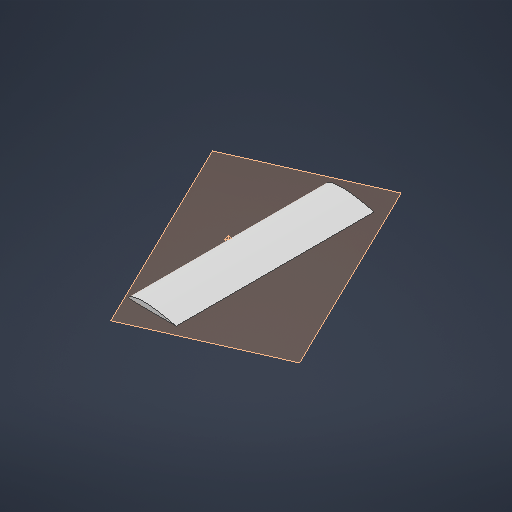
# Autodesk Inventor part: Airfoil
Saved by Autodesk Inventor 2026.1 (Build 301233000, 233)
## iProperties
Created: 2026-06-28
Part Number: Airfoil
Material: Generic
Document SubType Name: Modeling
Designer: adria
Density: 1 g/cm^3
Appearance: Default
Author: adria
Autodesk Inventor part; units mm, degrees
ref_plane "YZ Plane" through (0, 0, 0) normal (1, 0, 0) x (0, 1, 0)
ref_plane "XZ Plane" through (0, 0, 0) normal (0, 1, 0) x (-1, 0, 0)
ref_plane "XY Plane" through (0, 0, 0) normal (0, 0, 1) x (1, 0, 0)
sketch "Airfoil" plane through (0, 0, 0) normal (0, 0, 1) x (1, 0, 0)
  spline S0 degree 3 poles (360.0001, -3.1258) (359.9999, -3.1093) (358.5352, -2.9642) (357.0563, -2.6727) (353.499, -2.1006) (349.1715, -1.2943) (343.5455, -0.2589) (336.9185, 1.0019) (329.2813, 2.4997) (320.7437, 4.2061) (311.3885, 6.1167) (301.3069, 8.1831) (290.5978, 10.3802) (279.3545, 12.6643) (267.6408, 14.9381) (255.5164, 17.1385) (243.0539, 19.2958) (230.3132, 21.3308) (217.3729, 23.2252) (204.3064, 24.9736) (191.1725, 26.4966) (178.0452, 27.8241) (164.9837, 28.9046) (152.0591, 29.712) (139.3323, 30.2778) (126.8644, 30.5476) (114.7179, 30.5317) (102.9483, 30.2384) (91.6056, 29.6426) (80.7401, 28.7689) (70.3983, 27.6332) (60.634, 26.2223) (51.4811, 24.5969) (42.9826, 22.7423) (35.1746, 20.693) (28.0854, 18.4861) (21.7475, 16.1422) (16.1794, 13.7122) (11.405, 11.2286) (7.4429, 8.7282) (4.3064, 6.298) (1.9678, 3.9602) (0.5759, 1.8788) (-0.2825, -0.1229) (0.8182, -1.9616) (2.9085, -3.1846) (5.9423, -4.3926) (10.0909, -5.2147) (15.3188, -5.8919) (21.6524, -6.4415) (29.0414, -6.8802) (37.4377, -7.2114) (46.7843, -7.4502) (57.0133, -7.6106) (68.0506, -7.6971) (79.8194, -7.7126) (92.2551, -7.6326) (105.2911, -7.4608) (118.8533, -7.2529) (132.849, -7.0142) (147.1809, -6.7663) (161.7434, -6.5195) (176.4331, -6.2697) (191.1431, -6.0148) (205.7764, -5.7632) (220.2333, -5.52) (234.4223, -5.2741) (248.2526, -5.0368) (261.628, -4.8128) (274.4379, -4.5908) (286.5696, -4.3821) (297.9608, -4.1861) (308.5993, -4.0068) (318.4689, -3.8376) (327.5045, -3.6854) (335.6112, -3.5403) (342.6591, -3.4259) (348.6433, -3.3202) (353.2298, -3.2392) (356.964, -3.1905) (358.5007, -3.1269) (360.0002, -3.1425) (360.0001, -3.1258) knots 0 0 0 0 0.000951 0.003756 0.008317 0.014521 0.022293 0.03156 0.04222 0.054151 0.067231 0.081331 0.096307 0.112011 0.128327 0.145184 0.162487 0.180134 0.198032 0.216058 0.234133 0.25219 0.270102 0.287815 0.305233 0.322283 0.338894 0.354984 0.370504 0.385415 0.39963 0.413113 0.42582 0.437701 0.448735 0.458877 0.468103 0.476402 0.483746 0.490131 0.495554 0.500009 0.503513 0.506003 0.508226 0.511498 0.515852 0.521548 0.528758 0.537453 0.547579 0.559078 0.571871 0.585877 0.600983 0.617084 0.634085 0.651924 0.670487 0.689646 0.709262 0.729203 0.749306 0.769443 0.789468 0.809256 0.828671 0.847599 0.865917 0.883468 0.900079 0.915619 0.930136 0.943664 0.956051 0.96716 0.976853 0.984996 0.991473 0.996184 0.999041 1 1 1 1
  line L0 (360.0001, -3.1258) -> (359.9999, -3.1093) construction
  line L1 (359.9999, -3.1093) -> (358.5352, -2.9642) construction
  line L2 (358.5352, -2.9642) -> (357.0563, -2.6727) construction
  line L3 (357.0563, -2.6727) -> (353.499, -2.1006) construction
  line L4 (353.499, -2.1006) -> (349.1715, -1.2943) construction
  line L5 (349.1715, -1.2943) -> (343.5455, -0.2589) construction
  line L6 (343.5455, -0.2589) -> (336.9185, 1.0019) construction
  line L7 (336.9185, 1.0019) -> (329.2813, 2.4997) construction
  line L8 (329.2813, 2.4997) -> (320.7437, 4.2061) construction
  line L9 (320.7437, 4.2061) -> (311.3885, 6.1167) construction
  line L10 (311.3885, 6.1167) -> (301.3069, 8.1831) construction
  line L11 (301.3069, 8.1831) -> (290.5978, 10.3802) construction
  line L12 (290.5978, 10.3802) -> (279.3545, 12.6643) construction
  line L13 (279.3545, 12.6643) -> (267.6408, 14.9381) construction
  line L14 (267.6408, 14.9381) -> (255.5164, 17.1385) construction
  line L15 (255.5164, 17.1385) -> (243.0539, 19.2958) construction
  line L16 (243.0539, 19.2958) -> (230.3132, 21.3308) construction
  line L17 (230.3132, 21.3308) -> (217.3729, 23.2252) construction
  line L18 (217.3729, 23.2252) -> (204.3064, 24.9736) construction
  line L19 (204.3064, 24.9736) -> (191.1725, 26.4966) construction
  line L20 (191.1725, 26.4966) -> (178.0452, 27.8241) construction
  line L21 (178.0452, 27.8241) -> (164.9837, 28.9046) construction
  line L22 (164.9837, 28.9046) -> (152.0591, 29.712) construction
  line L23 (152.0591, 29.712) -> (139.3323, 30.2778) construction
  line L24 (139.3323, 30.2778) -> (126.8644, 30.5476) construction
  line L25 (126.8644, 30.5476) -> (114.7179, 30.5317) construction
  line L26 (114.7179, 30.5317) -> (102.9483, 30.2384) construction
  line L27 (102.9483, 30.2384) -> (91.6056, 29.6426) construction
  line L28 (91.6056, 29.6426) -> (80.7401, 28.7689) construction
  line L29 (80.7401, 28.7689) -> (70.3983, 27.6332) construction
  line L30 (70.3983, 27.6332) -> (60.634, 26.2223) construction
  line L31 (60.634, 26.2223) -> (51.4811, 24.5969) construction
  line L32 (51.4811, 24.5969) -> (42.9826, 22.7423) construction
  line L33 (42.9826, 22.7423) -> (35.1746, 20.693) construction
  line L34 (35.1746, 20.693) -> (28.0854, 18.4861) construction
  line L35 (28.0854, 18.4861) -> (21.7475, 16.1422) construction
  line L36 (21.7475, 16.1422) -> (16.1794, 13.7122) construction
  line L37 (16.1794, 13.7122) -> (11.405, 11.2286) construction
  line L38 (11.405, 11.2286) -> (7.4429, 8.7282) construction
  line L39 (7.4429, 8.7282) -> (4.3064, 6.298) construction
  line L40 (4.3064, 6.298) -> (1.9678, 3.9602) construction
  line L41 (1.9678, 3.9602) -> (0.5759, 1.8788) construction
  line L42 (0.5759, 1.8788) -> (-0.2825, -0.1229) construction
  line L43 (-0.2825, -0.1229) -> (0.8182, -1.9616) construction
  line L44 (0.8182, -1.9616) -> (2.9085, -3.1846) construction
  line L45 (2.9085, -3.1846) -> (5.9423, -4.3926) construction
  line L46 (5.9423, -4.3926) -> (10.0909, -5.2147) construction
  line L47 (10.0909, -5.2147) -> (15.3188, -5.8919) construction
  line L48 (15.3188, -5.8919) -> (21.6524, -6.4415) construction
  line L49 (21.6524, -6.4415) -> (29.0414, -6.8802) construction
  line L50 (29.0414, -6.8802) -> (37.4377, -7.2114) construction
  line L51 (37.4377, -7.2114) -> (46.7843, -7.4502) construction
  line L52 (46.7843, -7.4502) -> (57.0133, -7.6106) construction
  line L53 (57.0133, -7.6106) -> (68.0506, -7.6971) construction
  line L54 (68.0506, -7.6971) -> (79.8194, -7.7126) construction
  line L55 (79.8194, -7.7126) -> (92.2551, -7.6326) construction
  line L56 (92.2551, -7.6326) -> (105.2911, -7.4608) construction
  line L57 (105.2911, -7.4608) -> (118.8533, -7.2529) construction
  line L58 (118.8533, -7.2529) -> (132.849, -7.0142) construction
  line L59 (132.849, -7.0142) -> (147.1809, -6.7663) construction
  line L60 (147.1809, -6.7663) -> (161.7434, -6.5195) construction
  line L61 (161.7434, -6.5195) -> (176.4331, -6.2697) construction
  line L62 (176.4331, -6.2697) -> (191.1431, -6.0148) construction
  line L63 (191.1431, -6.0148) -> (205.7764, -5.7632) construction
  line L64 (205.7764, -5.7632) -> (220.2333, -5.52) construction
  line L65 (220.2333, -5.52) -> (234.4223, -5.2741) construction
  line L66 (234.4223, -5.2741) -> (248.2526, -5.0368) construction
  line L67 (248.2526, -5.0368) -> (261.628, -4.8128) construction
  line L68 (261.628, -4.8128) -> (274.4379, -4.5908) construction
  line L69 (274.4379, -4.5908) -> (286.5696, -4.3821) construction
  line L70 (286.5696, -4.3821) -> (297.9608, -4.1861) construction
  line L71 (297.9608, -4.1861) -> (308.5993, -4.0068) construction
  line L72 (308.5993, -4.0068) -> (318.4689, -3.8376) construction
  line L73 (318.4689, -3.8376) -> (327.5045, -3.6854) construction
  line L74 (327.5045, -3.6854) -> (335.6112, -3.5403) construction
  line L75 (335.6112, -3.5403) -> (342.6591, -3.4259) construction
  line L76 (342.6591, -3.4259) -> (348.6433, -3.3202) construction
  line L77 (348.6433, -3.3202) -> (353.2298, -3.2392) construction
  line L78 (353.2298, -3.2392) -> (356.964, -3.1905) construction
  line L79 (356.964, -3.1905) -> (358.5007, -3.1269) construction
  line L80 (358.5007, -3.1269) -> (360.0002, -3.1425) construction
  line L81 (360.0002, -3.1425) -> (360.0001, -3.1258) construction
  line L82 (0, 0) -> (360.0001, -3.1258) construction
  point P0 (179.3364, 5.2593)
sketch "Sketch1" plane through (0, 0, 0) normal (0, 0, 1) x (1, 0, 0)
  line L0 (0, 0) -> (0, -30) construction
  line L1 (0, -30) -> (300, -30) construction
  spline S0 degree 3 poles (359.8903, -9.4241) (359.8904, -9.4075) (358.4284, -9.2368) (356.9549, -8.9194) (353.4081, -8.2852) (349.0954, -7.4034) (343.4884, -6.2696) (336.8844, -4.8931) (329.2747, -3.2619) (320.7682, -1.4064) (311.4479, 0.6676) (301.4039, 2.91) (290.7349, 5.2942) (279.5333, 7.7746) (267.8612, 10.2531) (255.7771, 12.6653) (243.3543, 15.0402) (230.6512, 17.2979) (217.746, 19.4184) (204.712, 21.3951) (191.6068, 23.1477) (178.5047, 24.7047) (165.4642, 26.0136) (152.5557, 27.047) (139.8408, 27.8354) (127.3795, 28.3233) (115.2345, 28.5198) (103.4616, 28.4326) (92.1102, 28.0353) (81.2311, 27.3519) (70.8711, 26.3973) (61.0835, 25.1574) (51.9036, 23.6924) (43.374, 21.9868) (35.5313, 20.0744) (28.4046, 17.9919) (22.0266, 15.7592) (16.4168, 13.427) (11.5997, 11.0273) (7.5944, 8.5967) (4.4159, 6.2217) (2.0368, 3.9251) (0.6086, 1.8684) (-0.2846, -0.1179) (0.7837, -1.9756) (2.8523, -3.235) (5.8645, -4.4959) (9.9981, -5.3905) (15.2134, -6.159) (21.5363, -6.8193) (28.9165, -7.3873) (37.3058, -7.8653) (46.6468, -8.2676) (56.8714, -8.607) (67.9055, -8.8866) (79.6723, -9.108) (92.1074, -9.2455) (105.1444, -9.3019) (118.7082, -9.3313) (132.7059, -9.3375) (147.04, -9.3404) (161.6045, -9.3484) (176.2964, -9.3557) (191.0086, -9.3582) (205.644, -9.3627) (220.103, -9.3725) (234.2942, -9.3748) (248.1264, -9.3796) (261.5037, -9.3896) (274.3155, -9.3917) (286.4491, -9.3953) (297.842, -9.3987) (308.4819, -9.4056) (318.353, -9.4091) (327.3899, -9.415) (335.4978, -9.4117) (342.5467, -9.4207) (348.5319, -9.4197) (353.1191, -9.4189) (356.8535, -9.4356) (358.3911, -9.3989) (359.8902, -9.4407) (359.8903, -9.4241) knots 0 0 0 0 0.000951 0.003756 0.008317 0.014521 0.022293 0.03156 0.04222 0.054151 0.067231 0.081331 0.096307 0.112011 0.128327 0.145184 0.162487 0.180134 0.198032 0.216058 0.234133 0.25219 0.270102 0.287815 0.305233 0.322283 0.338894 0.354984 0.370504 0.385415 0.39963 0.413113 0.42582 0.437701 0.448735 0.458877 0.468103 0.476402 0.483746 0.490131 0.495554 0.500009 0.503513 0.506003 0.508226 0.511498 0.515852 0.521548 0.528758 0.537453 0.547579 0.559078 0.571871 0.585877 0.600983 0.617084 0.634085 0.651924 0.670487 0.689646 0.709262 0.729203 0.749306 0.769443 0.789468 0.809256 0.828671 0.847599 0.865917 0.883468 0.900079 0.915619 0.930136 0.943664 0.956051 0.96716 0.976853 0.984996 0.991473 0.996184 0.999041 1 1 1 1
  line L2 (359.8903, -9.4241) -> (359.8904, -9.4075) construction
  line L3 (359.8904, -9.4075) -> (358.4284, -9.2368) construction
  line L4 (358.4284, -9.2368) -> (356.9549, -8.9194) construction
  line L5 (356.9549, -8.9194) -> (353.4081, -8.2852) construction
  line L6 (353.4081, -8.2852) -> (349.0954, -7.4034) construction
  line L7 (349.0954, -7.4034) -> (343.4884, -6.2696) construction
  line L8 (343.4884, -6.2696) -> (336.8844, -4.8931) construction
  line L9 (336.8844, -4.8931) -> (329.2747, -3.2619) construction
  line L10 (329.2747, -3.2619) -> (320.7682, -1.4064) construction
  line L11 (320.7682, -1.4064) -> (311.4479, 0.6676) construction
  line L12 (311.4479, 0.6676) -> (301.4039, 2.91) construction
  line L13 (301.4039, 2.91) -> (290.7349, 5.2942) construction
  line L14 (290.7349, 5.2942) -> (279.5333, 7.7746) construction
  line L15 (279.5333, 7.7746) -> (267.8612, 10.2531) construction
  line L16 (267.8612, 10.2531) -> (255.7771, 12.6653) construction
  line L17 (255.7771, 12.6653) -> (243.3543, 15.0402) construction
  line L18 (243.3543, 15.0402) -> (230.6512, 17.2979) construction
  line L19 (230.6512, 17.2979) -> (217.746, 19.4184) construction
  line L20 (217.746, 19.4184) -> (204.712, 21.3951) construction
  line L21 (204.712, 21.3951) -> (191.6068, 23.1477) construction
  line L22 (191.6068, 23.1477) -> (178.5047, 24.7047) construction
  line L23 (178.5047, 24.7047) -> (165.4642, 26.0136) construction
  line L24 (165.4642, 26.0136) -> (152.5557, 27.047) construction
  line L25 (152.5557, 27.047) -> (139.8408, 27.8354) construction
  line L26 (139.8408, 27.8354) -> (127.3795, 28.3233) construction
  line L27 (127.3795, 28.3233) -> (115.2345, 28.5198) construction
  line L28 (115.2345, 28.5198) -> (103.4616, 28.4326) construction
  line L29 (103.4616, 28.4326) -> (92.1102, 28.0353) construction
  line L30 (92.1102, 28.0353) -> (81.2311, 27.3519) construction
  line L31 (81.2311, 27.3519) -> (70.8711, 26.3973) construction
  line L32 (70.8711, 26.3973) -> (61.0835, 25.1574) construction
  line L33 (61.0835, 25.1574) -> (51.9036, 23.6924) construction
  line L34 (51.9036, 23.6924) -> (43.374, 21.9868) construction
  line L35 (43.374, 21.9868) -> (35.5313, 20.0744) construction
  line L36 (35.5313, 20.0744) -> (28.4046, 17.9919) construction
  line L37 (28.4046, 17.9919) -> (22.0266, 15.7592) construction
  line L38 (22.0266, 15.7592) -> (16.4168, 13.427) construction
  line L39 (16.4168, 13.427) -> (11.5997, 11.0273) construction
  line L40 (11.5997, 11.0273) -> (7.5944, 8.5967) construction
  line L41 (7.5944, 8.5967) -> (4.4159, 6.2217) construction
  line L42 (4.4159, 6.2217) -> (2.0368, 3.9251) construction
  line L43 (2.0368, 3.9251) -> (0.6086, 1.8684) construction
  line L44 (0.6086, 1.8684) -> (-0.2846, -0.1179) construction
  line L45 (-0.2846, -0.1179) -> (0.7837, -1.9756) construction
  line L46 (0.7837, -1.9756) -> (2.8523, -3.235) construction
  line L47 (2.8523, -3.235) -> (5.8645, -4.4959) construction
  line L48 (5.8645, -4.4959) -> (9.9981, -5.3905) construction
  line L49 (9.9981, -5.3905) -> (15.2134, -6.159) construction
  line L50 (15.2134, -6.159) -> (21.5363, -6.8193) construction
  line L51 (21.5363, -6.8193) -> (28.9165, -7.3873) construction
  line L52 (28.9165, -7.3873) -> (37.3058, -7.8653) construction
  line L53 (37.3058, -7.8653) -> (46.6468, -8.2676) construction
  line L54 (46.6468, -8.2676) -> (56.8714, -8.607) construction
  line L55 (56.8714, -8.607) -> (67.9055, -8.8866) construction
  line L56 (67.9055, -8.8866) -> (79.6723, -9.108) construction
  line L57 (79.6723, -9.108) -> (92.1074, -9.2455) construction
  line L58 (92.1074, -9.2455) -> (105.1444, -9.3019) construction
  line L59 (105.1444, -9.3019) -> (118.7082, -9.3313) construction
  line L60 (118.7082, -9.3313) -> (132.7059, -9.3375) construction
  line L61 (132.7059, -9.3375) -> (147.04, -9.3404) construction
  line L62 (147.04, -9.3404) -> (161.6045, -9.3484) construction
  line L63 (161.6045, -9.3484) -> (176.2964, -9.3557) construction
  line L64 (176.2964, -9.3557) -> (191.0086, -9.3582) construction
  line L65 (191.0086, -9.3582) -> (205.644, -9.3627) construction
  line L66 (205.644, -9.3627) -> (220.103, -9.3725) construction
  line L67 (220.103, -9.3725) -> (234.2942, -9.3748) construction
  line L68 (234.2942, -9.3748) -> (248.1264, -9.3796) construction
  line L69 (248.1264, -9.3796) -> (261.5037, -9.3896) construction
  line L70 (261.5037, -9.3896) -> (274.3155, -9.3917) construction
  line L71 (274.3155, -9.3917) -> (286.4491, -9.3953) construction
  line L72 (286.4491, -9.3953) -> (297.842, -9.3987) construction
  line L73 (297.842, -9.3987) -> (308.4819, -9.4056) construction
  line L74 (308.4819, -9.4056) -> (318.353, -9.4091) construction
  line L75 (318.353, -9.4091) -> (327.3899, -9.415) construction
  line L76 (327.3899, -9.415) -> (335.4978, -9.4117) construction
  line L77 (335.4978, -9.4117) -> (342.5467, -9.4207) construction
  line L78 (342.5467, -9.4207) -> (348.5319, -9.4197) construction
  line L79 (348.5319, -9.4197) -> (353.1191, -9.4189) construction
  line L80 (353.1191, -9.4189) -> (356.8535, -9.4356) construction
  line L81 (356.8535, -9.4356) -> (358.3911, -9.3989) construction
  line L82 (358.3911, -9.3989) -> (359.8902, -9.4407) construction
  line L83 (359.8902, -9.4407) -> (359.8903, -9.4241) construction
  line L84 (0, 0) -> (359.8903, -9.4241) construction
  point P0 (0, 0)
  dimension "d4" = 30
  dimension "d5" = 300
  dimension "d6" = -1.5
  constraints: 4 end point, 1 horizontal, 1 vertical, 2 other
  measures "d4" distance of L0.start L0.end
  measures "d5" distance of L0.end L1.end
extrude "Extrusion1" add sketch "Sketch1" along normal mid plane 1500
ref_plane "Work Plane1" through (0, 0, 0) normal (0.0261769, 0.9996573, 0) x (0.4325961, -0.0113279, 0.9015167)
body "Solid1"
